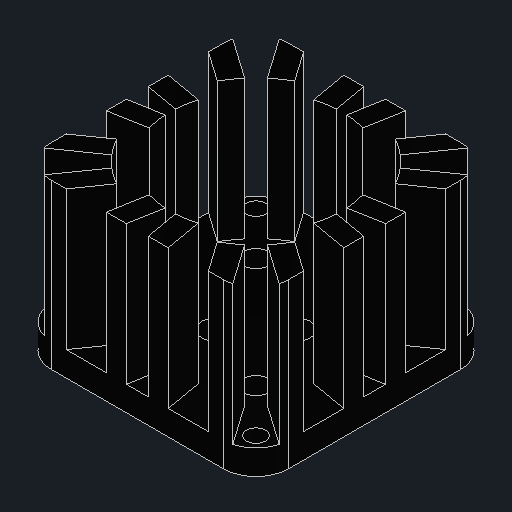
# Autodesk Inventor part: 680-125K
Saved by Autodesk Inventor 2026.3 (Build 303398000, 398)
## iProperties
Created: 2026-05-22
Part Number: 680-125K
Material: Aluminum-5052
Document SubType Name: Modeling
Designer: JGW
Mass: 58.7182 g
Surface Area: 152.224 cm^2
Volume: 21.6672 cm^3
Density: 2.71 g/cm^3
Appearance: Anodized - Black
CurrentECO: -
Author: JGW
Autodesk Inventor part; units mm, degrees
ref_plane "YZ Plane" through (0, 0, 0) normal (1, 0, 0) x (0, 1, 0)
ref_plane "XZ Plane" through (0, 0, 0) normal (0, 1, 0) x (-1, 0, 0)
sketch "Sketch2" plane through (0, 0, 0) normal (0, 1, 0) x (-1, 0, 0)
  line L0 (23, 23) -> (-23, 23)
  line L1 (-23, 23) -> (-23, -23)
  line L2 (-23, -23) -> (23, -23)
  line L3 (23, -23) -> (23, 23)
  line L4 (23, 23) -> (-23, -23) construction
  line L5 (-23, 23) -> (23, -23) construction
  circle A0 centre (19.05, -19.05) radius 1.8669
  line L6 (0, -32.2) -> (0, 32.2) construction
  line L7 (-32.2, 0) -> (32.2, 0) construction
  circle A1 centre (-19.05, -19.05) radius 1.8669
  circle A2 centre (19.05, 19.05) radius 1.8669
  circle A3 centre (-19.05, 19.05) radius 1.8669
  circle A4 centre (-5.1187, -2.6043) radius 2.794
  circle A5 centre (2.6043, 5.1187) radius 2.794
  circle A6 centre (10.6604, -10.6604) radius 2.413
  circle A7 centre (-10.6604, 10.6604) radius 2.413
  line L8 (2.6043, 5.1187) -> (-5.1187, -2.6043) construction
  point P0 (0, 0)
  point P1 (-1.2572, 1.2572)
  dimension "d4" = 46
  dimension "d5" = 46
  dimension "d8" = 38.1
  dimension "d11" = 38.1
  dimension "d14" = 3.7338
  dimension "d15" = 5.588
  dimension "d16" = 4.826
  dimension "d17" = 30.1521
  dimension "d18" = 15.0761
  dimension "d19" = 10.922
  dimension "d20" = 1.778
  constraints: 14 end point, 8 centre point, 3 midpoint, 3 parallel, 3 point on line, 2 equal radius, 2 horizontal, 2 symmetric about line, 1 perpendicular, 1 vertical, 6 other
  measures "d4" distance of L2.end L1.end
  measures "d5" distance of L1.end L0.end
  measures "d8" distance of A0.centre A1.centre
  measures "d11" distance of A0.centre A2.centre
  measures "d14" diameter of A2
  measures "d15" diameter of A5
  measures "d16" diameter of A6
  measures "d17" distance of A7.centre A6.centre
  measures "d18" distance from line of L4 A6.centre
  measures "d19" distance of L8.end L8.start
  measures "d20" distance between parallel lines of L4 L8
extrude "Extrusion1" add sketch "Sketch2" along normal blind 31.75 contours L3 L2 L1 L0 | A0 | A1 | A2 | A3 | A4 | A5 | A6 | A7
fillet "Fillet1" radius 6.35 4 edges at (-23, 15.875, 23) (-23, 15.875, -23) (23, 15.875, 23) (23, 15.875, -23)
ref_plane "Work Plane1" through (0, 4.7752, 0) normal (0, -1, 0) x (1, 0, 0)
sketch "Sketch3" plane through (0, 4.7752, 0) normal (0, -1, 0) x (1, 0, 0)
  circle A0 centre (0, 0) radius 19.812
  circle A1 centre (0, 0) radius 16.637
  line L0 (23, 16.65) -> (23, -16.65) construction
  line L1 (23, -5.9899) -> (15.9457, -4.746)
  line L2 (16.6073, -0.9939) -> (23, -2.1211)
  line L3 (16.6073, 0.9939) -> (23, 2.1211)
  line L4 (15.9457, 4.746) -> (23, 5.9899)
  line L5 (-36.211, 0) -> (36.9584, 0) construction
  line L6 (16.3842, -2.889) -> (23, -4.0555) construction
  line L7 (23, -2.1211) -> (23, 2.1211)
  line L8 (9.7506, -17.2465) -> (13.7792, -23)
  line L9 (16.65, -23) -> (-16.65, -23) construction
  line L10 (18.4303, -23) -> (12.8715, -15.0612)
  line L11 (15.0612, -12.8715) -> (23, -18.4303)
  line L12 (17.2465, -9.7506) -> (23, -13.7792)
  line L13 (0, 36.211) -> (0, -36.9584) construction
  line L14 (0, 0) -> (26.5056, -26.5056) construction
  line L15 (16.1048, -23) -> (11.3637, -16.229) construction
  arc A2 (18.4303, -23) -> (23, -18.4303) centre (21.1181, -21.1181) ccw
  line L16 (23, -13.7792) -> (23, -5.9899)
  line L17 (0.9939, 16.6073) -> (2.1211, 23)
  line L18 (5.9899, 23) -> (4.746, 15.9457)
  line L19 (2.1211, 23) -> (-2.1211, 23)
  line L20 (-0.9939, 16.6073) -> (-2.1211, 23)
  line L21 (-4.746, 15.9457) -> (-5.9899, 23)
  line L22 (13.7792, 23) -> (5.9899, 23)
  line L23 (9.7506, 17.2465) -> (13.7792, 23)
  line L24 (12.8715, 15.0612) -> (18.4303, 23)
  line L25 (23, 18.4303) -> (15.0612, 12.8715)
  line L26 (17.2465, 9.7506) -> (23, 13.7792)
  arc A3 (23, 18.4303) -> (18.4303, 23) centre (21.1181, 21.1181) ccw
  line L27 (-16.6073, 0.9939) -> (-23, 2.1211)
  line L28 (-23, 5.9899) -> (-15.9457, 4.746)
  line L29 (-23, 2.1211) -> (-23, -2.1211)
  line L30 (-16.6073, -0.9939) -> (-23, -2.1211)
  line L31 (-15.9457, -4.746) -> (-23, -5.9899)
  line L32 (-23, 13.7792) -> (-23, 5.9899)
  line L33 (-17.2465, 9.7506) -> (-23, 13.7792)
  line L34 (-15.0612, 12.8715) -> (-23, 18.4303)
  line L35 (-18.4303, 23) -> (-12.8715, 15.0612)
  line L36 (-9.7506, 17.2465) -> (-13.7792, 23)
  arc A4 (-18.4303, 23) -> (-23, 18.4303) centre (-21.1181, 21.1181) ccw
  line L37 (-0.9939, -16.6073) -> (-2.1211, -23)
  line L38 (-5.9899, -23) -> (-4.746, -15.9457)
  line L39 (-2.1211, -23) -> (2.1211, -23)
  line L40 (0.9939, -16.6073) -> (2.1211, -23)
  line L41 (4.746, -15.9457) -> (5.9899, -23)
  line L42 (-13.7792, -23) -> (-5.9899, -23)
  line L43 (-9.7506, -17.2465) -> (-13.7792, -23)
  line L44 (-12.8715, -15.0612) -> (-18.4303, -23)
  line L45 (-23, -18.4303) -> (-15.0612, -12.8715)
  line L46 (-17.2465, -9.7506) -> (-23, -13.7792)
  arc A5 (-23, -18.4303) -> (-18.4303, -23) centre (-21.1181, -21.1181) ccw
  line L47 (23, 5.9899) -> (23, 13.7792)
  line L48 (-5.9899, 23) -> (-13.7792, 23)
  line L49 (-23, -5.9899) -> (-23, -13.7792)
  line L50 (-23, -16.65) -> (-23, 16.65) construction
  line L51 (13.7792, -23) -> (5.9899, -23)
  point P0 (19.0898, 5.3004)
  dimension "d25" = 39.624
  dimension "d26" = 33.274
  dimension "d27" = 3.81
  dimension "d28" = 3.81
  dimension "d29" = 20
  dimension "d30" = 45
  dimension "d31" = 3.81
  dimension "d32" = 3.81
  dimension "d33" = 20
  dimension "d41" = 360
  constraints: 94 end point, 18 point on circle, 6 centre point, 5 point on line, 4 parallel, 3 vertical, 2 coincident, 2 collinear, 1 perpendicular, 1 tangent, 125 other
  measures "d25" diameter of A0
  measures "d26" diameter of A1
  measures "d27" distance between parallel lines of L2 L1
  measures "d28" distance between parallel lines of L4 L3
  measures "d29" angle of L3 L2
  measures "d30" angle of L5 L14
  measures "d31" distance between parallel lines of L10 L8
  measures "d32" distance between parallel lines of L12 L11
  measures "d33" angle of L11 L10
extrude "Extrusion2" cut sketch "Sketch3" against normal blind 31.75 contours A0 L4 A1 L18 | L26 L47 L4 A0 | A0 L24 A3 L25 | L3 L7 L2 A0 | A0 L2 A1 L3 | A1 | A0 L18 L22 L23 | A1 L20 A0 L17 | A0 L20 L19 L17 | L1 L16 L12 A0 | A0 L41 A1 L1 | A1 L28 A0 L21 | A0 L36 L48 L21 | L11 A2 L10 A0 | L40 A0 L37 A1 | A0 L8 L51 L41 | A1 L30 A0 L27 | L28 L32 L33 A0 | A0 L34 A4 L35 | L40 L39 L37 A0 | A0 L30 L29 L27 | L38 A0 L31 A1 | L38 L42 L43 A0 | A0 L46 L49 L31 | L44 A5 L45 A0
extrude "Extrusion3" cut sketch "Sketch2" along normal through all contours A0 | A1 | A2 | A3 | A4 | A5 | A6 | A7
equation "\"d18\" = 0.5 * d17"
equation "\"d28\" = d27"
equation "\"d31\" = d27"
equation "\"d32\" = d27"
body "Solid1"
